Roller (Autodesk Fusion 360 design; units mm, degrees)
part number: 2026-09-21-20-24-42-214
part number: 2026-09-23-19-50-07-162
Autodesk Fusion 360 part; units mm, degrees
sketch "Sketch3" plane through (0, 0, 0) normal (0, 0, 1) x (1, 0, 0)
  line L0 (-75, 25) -> (-25, 25)
  line L1 (-55, 35) -> (-55, 31)
  line L2 (-74, 35) -> (-74, 31)
  line L3 (-74, 31) -> (-71, 31)
  line L4 (-71, 31) -> (-71, 27)
  line L5 (-55, 31) -> (-58, 31)
  line L6 (-71, 27) -> (-58, 27)
  line L7 (-58, 27) -> (-58, 31)
  spline S0 degree 2 poles (-74, 35) (-64.5061, 38.8829) (-55, 35) knots 0 0 0 1.987265 1.987265 1.987265 weights 1 3 1
  dimension "d6" = 4
  constraint horizontal L0
  constraint parallel L1 L2
  constraint perpendicular L2 L3
  constraint perpendicular L3 L4
  constraint perpendicular L1 L5
  constraint perpendicular L4 L6
  constraint perpendicular L5 L7
  measures "d6" distance of L3.end L4.end
revolve "Revolve2" add sketch "Sketch3" angle 360 about axis through (-75, 25, 0) along (1, 0, 0) makes body 1
copy_body "Body->Comp1" bodies 1 removing the originals makes body 2 in component "Component"
sketch "Sketch1" plane through (0, 0, 0) normal (0, 0, 1) x (1, 0, 0)
  line L0 (-50, 30) -> (33.79, 30)
  line L1 (-50, 38) -> (-47, 38)
  line L2 (-47, 38) -> (-47, 34)
  line L3 (-47, 34) -> (20.1469, 34)
  line L4 (20.1469, 34) -> (20.1469, 38)
  line L5 (20.1469, 38) -> (23.1469, 38)
  line L6 (23.1469, 38) -> (23.1469, 42)
  line L7 (-50, 42) -> (-50, 38)
  spline S0 degree 2 poles (-50, 42) (-12, 57) (23.1469, 42) knots 0 0 0 7.653179 7.653179 7.653179 weights 1 3 1
  dimension "d1" = 83.79
  dimension "d2" = 90
  dimension "d3" = 3
  constraint horizontal L0
  constraint perpendicular L1 L2
  constraint perpendicular L1 L4
  constraint perpendicular L4 L5
  constraint perpendicular L5 L6
  constraint perpendicular L1 L7
  measures "d1" distance of L0.start L0.end
  measures "d2" angle of L2 L3
  measures "d3" distance of L4.end L5.end
revolve "Revolve1" [rolled back] along angle 360
sketch "Sketch2" plane through (0, 0, 0) normal (0, 0, 1) x (1, 0, 0)
component "Component" placed x (1, 0, 0) y (0, 1, 0) z (0, 0, 1) at (0, 0, 0)
